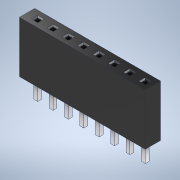
# Autodesk Inventor part: 8Pin_Header
Saved by Autodesk Inventor 2022 (Build 260153000, 153)
## iProperties
Created: 2022-12-26
Part Number: 8Pin_Header
Material: Generic
Document SubType Name: Modeling
Designer: karpova
Density: 1 g/cm^3
Appearance: PTFE
Author: karpova
Autodesk Inventor part; units mm, degrees
ref_plane "YZ Plane" through (0, 0, 0) normal (1, 0, 0) x (0, 1, 0)
ref_plane "XZ Plane" through (0, 0, 0) normal (0, 1, 0) x (-1, 0, 0)
ref_plane "XY Plane" through (0, 0, 0) normal (0, 0, 1) x (1, 0, 0)
sketch "Sketch1" plane through (0, 0, 0) normal (0, 0, 1) x (1, 0, 0)
  line L0 (-10.41, -2.0768) -> (10.41, -2.0768)
  line L1 (10.41, -2.0768) -> (10.41, 6.4232)
  line L2 (10.41, 6.4232) -> (-10.41, 6.4232)
  line L3 (-10.41, 6.4232) -> (-10.41, -2.0768)
  line L4 (0, 0) -> (0, 6.4232) construction
  dimension "d1" = 20.82
  dimension "d2" = 8.5
  constraints: 10 end point, 2 parallel, 1 horizontal, 1 midpoint, 1 perpendicular, 1 vertical, 1 other
  measures "d1" distance of L1.end L2.end
  measures "d2" distance of L0.end L1.end
extrude "Extrusion1" add sketch "Sketch1" along normal blind 2.54
sketch "Sketch3" plane through (-10.41, 6.4232, 0) normal (0, 1, 0) x (1, 0, 0)
  line L0 (0, 0) -> (0, -2.54) construction
  line L1 (0, -1.27) -> (20.82, -1.27) construction
  line L2 (20.82, 0) -> (20.82, -2.54) construction
  line L3 (19.2325, -0.9525) -> (19.8675, -0.9525)
  line L4 (19.8675, -0.9525) -> (19.8675, -1.5875)
  line L5 (19.8675, -1.5875) -> (19.2325, -1.5875)
  line L6 (19.2325, -1.5875) -> (19.2325, -0.9525)
  line L7 (19.55, -1.5875) -> (19.55, -0.9525) construction
  point P0 (10.41, 0)
  dimension "d18" = 0.635
  dimension "d19" = 1.27
  constraints: 12 end point, 4 midpoint, 2 parallel, 2 perpendicular, 1 horizontal, 1 other
  measures "d18" distance of L3.start L3.end
  measures "d19" distance between parallel lines of L2 L7
extrude "Extrusion3" cut sketch "Sketch3" against normal blind 6
chamfer "Chamfer1" distance 0.2 angle 45 4 edges at (8.8225, 6.4232, 1.27) (9.14, 6.4232, 0.9525) (9.4575, 6.4232, 1.27) (9.14, 6.4232, 1.5875)
pattern_linear "Rectangular Pattern1" count 8 spacing 2.54 along (-1, 0, 0) of "Extrusion3", "Chamfer1"
sketch "Sketch4" plane through (-10.41, -2.0768, 0) normal (0, -1, 0) x (1, 0, 0)
  line L0 (19.2325, 1.5875) -> (19.8675, 1.5875)
  line L1 (19.8675, 1.5875) -> (19.8675, 0.9525)
  line L2 (19.8675, 0.9525) -> (19.2325, 0.9525)
  line L3 (19.2325, 0.9525) -> (19.2325, 1.5875)
  line L4 (0, 0) -> (0, 2.54) construction
  line L5 (0, 1.27) -> (20.82, 1.27) construction
  line L6 (20.82, 0) -> (20.82, 2.54) construction
  line L7 (19.55, 0.9525) -> (19.55, 1.5875) construction
  point P0 (10.41, 0)
  dimension "d28" = 0.635
  dimension "d29" = 1.27
  constraints: 12 end point, 4 midpoint, 2 horizontal, 2 parallel, 2 perpendicular, 1 other
  measures "d28" distance of L0.end L1.end
  measures "d29" distance between parallel lines of L6 L7
extrude "Extrusion4" add sketch "Sketch4" along normal blind 3.2
chamfer "Chamfer2" distance 0.2 angle 45 4 edges at (8.8225, -5.2768, 1.27) (9.14, -5.2768, 1.5875) (9.4575, -5.2768, 1.27) (9.14, -5.2768, 0.9525)
pattern_linear "Rectangular Pattern2" count 8 spacing 2.54 along (-1, 0, 0) of "Extrusion4", "Chamfer2"
equation "\"d22\" = pinChamfer"
equation "\"d32\" = pinChamfer"
equation "\"pinChamfer\" = 0.2"
body "Solid1"
